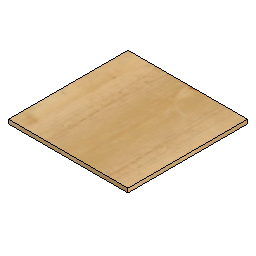
vaccine box model_ (Autodesk Fusion 360 archive; units mm, degrees)
design "dhakkan 2"
part number: 2025-11-06-22-35-00-341
Autodesk Fusion 360 part; units mm, degrees
sketch "Sketch1" plane through (0, 0, 0) normal (0, 0, 1) x (1, 0, 0)
  line L0 (0, 0) -> (322, 0)
  line L1 (322, 0) -> (322, 322)
  line L2 (322, 322) -> (0, 322)
  line L3 (0, 322) -> (0, 0)
  dimension "d1" = 322
  dimension "d2" = 322
  constraint horizontal L0
  constraint vertical L1
  constraint horizontal L2
  constraint vertical L3
  constraint coincident L0.start L3.end
  measures "d1" distance of L0.start L0.end
  measures "d2" distance of L0.start L2.end
extrude "Extrude1" add sketch "Sketch1" against normal blind 11
sketch "Sketch2" plane through (0, 0, -11) normal (0, 0, -1) x (1, 0, 0)
  line L0 (0, 0) -> (0, -322)
  line L1 (0, -322) -> (322, -322)
  line L2 (322, -322) -> (322, 0)
  line L3 (322, 0) -> (0, 0)
  line L4 (41, -41) -> (279.137, -41)
  line L5 (279.137, -41) -> (279.137, -280.7037)
  line L6 (279.137, -280.7037) -> (41, -280.7037)
  line L7 (41, -280.7037) -> (41, -41)
  dimension "d7" = 41
  dimension "d8" = 41
  constraint horizontal L4
  constraint vertical L5
  constraint horizontal L6
  constraint vertical L7
  measures "d7" distance of L3 L4
  measures "d8" distance of L0 L7
extrude "Extrude2" add sketch "Sketch2" along normal blind 30 contours L4 L5 L6 L7
